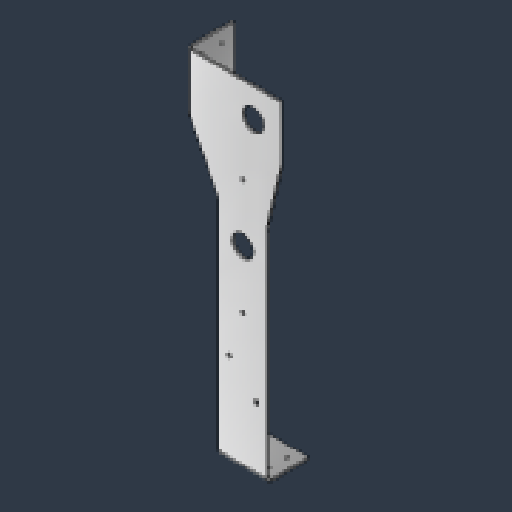
# Autodesk Inventor part: feeder_guide_plate
Saved by Autodesk Inventor 2024.3 (Build 283343000, 343)
## iProperties
Created: 2025-03-08
Part Number: feeder_guide_plate
Material: Aluminum 6061
Document SubType Name: Sheet Metal
Designer: marcu
Density: 2.7 g/cm^3
Sheet Metal Rule: Default
Appearance: Aluminum - Flat
Author: marcu
Autodesk Inventor part; units mm, degrees
ref_plane "YZ Plane" through (0, 0, 0) normal (1, 0, 0) x (0, 1, 0)
ref_plane "XZ Plane" through (0, 0, 0) normal (0, 1, 0) x (-1, 0, 0)
ref_plane "XY Plane" through (0, 0, 0) normal (0, 0, 1) x (1, 0, 0)
sketch "Sketch1" plane through (0, 0, 0) normal (0, 0, 1) x (1, 0, 0)
  line L0 (31.75, -147.6375) -> (-31.75, -147.6375)
  line L1 (-31.75, -147.6375) -> (-31.75, 147.6375)
  line L2 (-31.75, 147.6375) -> (31.75, 147.6375) construction
  line L3 (31.75, 147.6375) -> (31.75, -147.6375)
  line L4 (31.75, -147.6375) -> (-31.75, 147.6375) construction
  line L5 (-31.75, -147.6375) -> (31.75, 147.6375) construction
  line L6 (31.75, 147.6375) -> (49.2125, 223.8375)
  line L7 (-31.75, 147.6375) -> (-31.75, 300.0375) construction
  line L8 (-31.75, 300.0375) -> (49.2125, 300.0375)
  line L9 (49.2125, 223.8375) -> (49.2125, 300.0375)
  line L10 (-31.75, 300.0375) -> (-69.85, 300.0375)
  line L11 (-69.85, 300.0375) -> (-69.85, 223.8375)
  line L12 (-69.85, 223.8375) -> (-31.75, 223.8375) construction
  line L13 (-31.75, 223.8375) -> (-31.75, 300.0375) construction
  line L14 (-69.85, 223.8375) -> (-31.75, 147.6375)
  point P0 (0, 0)
  dimension "d0" = 63.5
  dimension "d1" = 295.275
  dimension "d2" = 80.9625
  dimension "d3" = 152.4
  dimension "d43" = 76.2
  dimension "d63" = 38.1
  dimension "d64" = 76.2
  measures "d0" distance of L1.end L2.end
  measures "d1" distance of L0.end L1.end
  measures "d2" distance from line of L8.end L1
  measures "d3" distance from line of L2 L8.end
  measures "d43" distance from line of L2 L6.end
  measures "d63" distance of L12.end L11.end
  measures "d64" distance of L11.end L10.end
extrude "Plate1" add sketch "Sketch1" along normal blind 3.175
sketch "Sketch2" plane through (0, 0, 3.175) normal (0, 0, 1) x (1, 0, 0)
  line L0 (31.75, -147.6375) -> (-31.75, -147.6375) construction
  line L1 (-31.75, -147.6375) -> (-31.75, 147.6375) construction
  line L2 (0, 109.7915) -> (13.3047, 261.8646) construction
  line L3 (0, 109.7915) -> (152.654, 109.7915) construction
  point P0 (0, 0)
  point P1 (0, -42.8625)
  point P2 (0, -147.6375)
  point P3 (-31.75, 300.0375)
  dimension "d5" = 104.775
  dimension "d8" = 152.654
  dimension "d29" = 31.75
  dimension "d98" = 152.654
  dimension "d99" = 85
  constraints: 4 end point, 1 coincident, 1 equal length, 1 horizontal, 1 midpoint, 1 vertical, 1 other
  measures "d5" distance from line of L0 point (0, -42.863)
  measures "d8" distance of point (0, -42.863) L2.start
  measures "d29" distance from line of L1 point (0, -42.863)
  measures "d98" distance of L2.start L2.end
  measures "d99" angle of L3 L2
hole "Hole1" at (0, 109.7915, 3.175) at (13.3047, 261.8646, 3.175) direction (0, 0, -1) diameter 28.575 end through all
sketch "Sketch3" plane through (0, 0, 3.175) normal (0, 0, 1) x (1, 0, 0)
  circle A0 centre (0, 109.7915) radius 14.2875 construction
  circle A1 centre (0, -42.8625) radius 14.2875 construction
  line L0 (0, 109.7915) -> (0, -42.8625) construction
  circle A2 centre (0, 262.4455) radius 14.2875 construction
  line L1 (0, 109.7915) -> (0, 262.4455) construction
  point P0 (0, 0)
  point P1 (0, 186.1185)
  point P2 (0, 33.4645)
  constraints: 4 end point, 2 midpoint, 2 vertical
hole "Hole2" at (0, 33.4645, 3.175) at (0, 186.1185, 3.175) direction (0, 0, -1) diameter 5.1054 end through all clearance for "Flat Head Machine Screw (82)" size "#10" standard "Ansi Unified Screw Threads"
fillet "Corner Round1" radius 50.8 1 edges at (31.75, 147.6375, 1.5875)
sketch "Sketch5" plane through (-31.75, -144.4625, 3.175) normal (0, -1, 0) x (1, 0, 0)
  line L0 (63.5, 0) -> (0, 0)
  line L1 (0, 0) -> (0, -55.5625)
  line L2 (0, -55.5625) -> (63.5, -55.5625)
  line L3 (63.5, -55.5625) -> (63.5, 0)
  constraints: 6 end point, 1 horizontal, 1 perpendicular, 1 vertical
edge flange "Flange2" height 52.3875 angle 90 thickness 3.175 bend radius 3.175 thickness toward (0, -1, 0) relief straight relief width 3.175 relief depth 1.5875 edges at (0, -147.6375, 0) wall of the first edge with corners at (31.75, -144.4625, 3.175) (-31.75, -144.4625, 3.175) (-31.75, -144.4625, -52.3875) (31.75, -144.4625, -52.3875)
bend "Bend2"
corner "Corner2"
sketch "Sketch6" plane through (0, 0, 3.175) normal (0, 0, 1) x (1, 0, 0)
  circle A0 centre (0, -42.8625) radius 14.2875 projected
  circle A1 centre (0, -42.8625) radius 25.4 construction
  line L0 (-17.9605, -24.902) -> (17.9605, -60.823) construction
  line L1 (0, -17.4625) -> (0, -68.2625) construction
  point P0 (0, 0)
  dimension "d54" = 50.8
  dimension "d55" = 45
  constraints: 4 end point, 4 point on circle, 3 coincident, 2 midpoint, 1 centre point, 1 vertical
  measures "d54" diameter of A1
  measures "d55" angle of L1 L0
hole "Hole3" at (-17.9605, -24.902, 3.175) at (17.9605, -60.823, 3.175) direction (0, 0, -1) diameter 6.35 end through all
sketch "Sketch7" plane through (-73.025, 300.0375, -3.175) normal (-1, 0, 0) x (0, -1, 0)
  line L0 (76.2, 0) -> (0, 0)
  line L1 (0, 0) -> (0, -55.5625)
  line L2 (0, -55.5625) -> (76.2, -55.5625)
  line L3 (76.2, -55.5625) -> (76.2, 0)
  constraints: 6 end point, 1 horizontal, 1 perpendicular, 1 vertical
edge flange "Flange3" height 61.9125 angle 90 thickness 3.175 bend radius 3.175 thickness toward (-1, 0, 0) relief straight relief width 3.175 relief depth 1.5875 edges at (-69.85, 261.9375, 0) wall of the first edge with corners at (-73.025, 223.8375, -3.175) (-73.025, 300.0375, -3.175) (-73.025, 300.0375, -58.7375) (-73.025, 223.8375, -58.7375)
bend "Bend3"
corner "Corner3"
sketch "Sketch8" plane through (-76.2, 223.8375, -58.7375) normal (-1, 0, 0) x (0, 0, 1)
  line L0 (0, 76.2) -> (55.5625, 76.2) projected
  line L1 (0, 0) -> (0, 76.2) projected
  point P0 (58.7375, -223.8375)
  point P1 (44.45, 60.325)
  point P2 (44.45, 15.875)
  point P3 (15.875, 15.875)
  point P4 (15.875, 60.325)
  dimension "d75" = 44.45
  dimension "d76" = 28.575
  dimension "d77" = 15.875
  dimension "d78" = 15.875
  constraints: 2 horizontal alignment, 2 vertical alignment
  measures "d75" distance of point (15.875, 15.875) point (15.875, 60.325)
  measures "d76" distance of point (44.45, 60.325) point (15.875, 60.325)
  measures "d77" distance from line of L0 point (15.875, 60.325)
  measures "d78" distance from line of L1 point (15.875, 60.325)
hole "Hole4" at (-76.2, 284.1625, -14.2875) at (-76.2, 239.7125, -14.2875) at (-76.2, 239.7125, -42.8625) at (-76.2, 284.1625, -42.8625) direction (1, 0, 0) diameter 5.1054 end through all
sketch "Sketch9" plane through (-31.75, -147.6375, -52.3875) normal (0, -1, 0) x (1, 0, 0)
  line L0 (0, 0) -> (0, 49.2125) projected
  line L1 (0, 55.5625) -> (63.5, 55.5625) projected
  line L2 (63.5, 0) -> (0, 0) projected
  point P0 (31.75, 52.3875)
  point P1 (14.2875, 39.6875)
  point P2 (49.2125, 39.6875)
  point P3 (49.2125, 14.2875)
  point P4 (14.2875, 14.2875)
  dimension "d86" = 14.2875
  dimension "d87" = 25.4
  dimension "d88" = 34.925
  dimension "d90" = 14.2875
  constraints: 2 horizontal alignment, 2 vertical alignment
  measures "d86" distance from line of L0 point (14.287, 39.688)
  measures "d87" distance of point (14.287, 39.688) point (14.287, 14.287)
  measures "d88" distance of point (49.212, 39.688) point (14.287, 39.688)
  measures "d90" distance from line of L2 point (14.287, 14.287)
hole "Hole5" at (-17.4625, -147.6375, -12.7) at (17.4625, -147.6375, -12.7) at (17.4625, -147.6375, -38.1) at (-17.4625, -147.6375, -38.1) direction (0, 1, 0) diameter 5.1054 end through all
equation "\"d18\" = Thickness"
equation "\"d61\" = Thickness"
equation "\"d78\" = d77"
equation "\"d84\" = Thickness"
equation "\"d4\" = Thickness"
equation "\"d44\" = BendReliefWidth"
equation "\"d45\" = BendReliefDepth"
equation "\"d46\" = MinimumRemnant"
equation "\"d47\" = TransitionRadius"
equation "\"d50\" = BendRadius"
equation "\"d51\" = CornerReliefSize"
equation "\"d52\" = GapSize"
equation "\"d53\" = JacobiRadiusSize"
equation "\"d65\" = BendReliefWidth"
equation "\"d66\" = BendReliefDepth"
equation "\"d67\" = MinimumRemnant"
equation "\"d68\" = TransitionRadius"
equation "\"d71\" = BendRadius"
equation "\"d72\" = CornerReliefSize"
equation "\"d73\" = GapSize"
equation "\"d74\" = JacobiRadiusSize"
equation "\"d90\" = d86"
equation "\"BendRadius\" = Thickness"
equation "\"BendReliefWidth\" = Thickness"
equation "\"BendReliefDepth\" = 0.5 * Thickness"
equation "\"CornerReliefSize\" = 4 * Thickness"
equation "\"MinimumRemnant\" = 2 * Thickness"
equation "\"TransitionRadius\" = BendRadius"
equation "\"JacobiRadiusSize\" = BendRadius"
equation "\"GapSize\" = Thickness"
equation "\"Thickness\" = 3.175"
body "Solid1"
